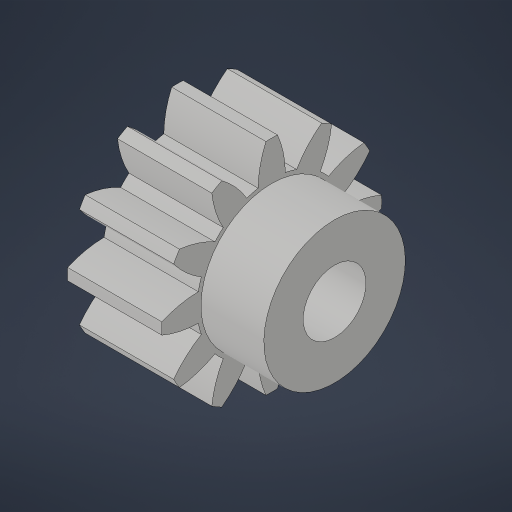
# Autodesk Inventor part: DS0.5-12_On
Saved by Autodesk Inventor 2024.2 (Build 282272000, 272)
## iProperties
Category: PARTsolutions
Company: KHK
Created: 2024-02-14
Part Number: DS0.5-12_On
Material: Generic
Catalog Web Link: www.cadenas.de
Description: Injection Molded Spur Gears (DS)-
Vendor: KHK
Document SubType Name: Modeling
Designer: psAdmin
Manufacturer: KHK
Mass: 0.117451 g
Surface Area: 2.6496 cm^2
Volume: 0.117451 cm^3
Density: 1 g/cm^3
Appearance: PSOLRGB-175-175-175
PSOL_IDENT_0: {$CADENAS_DATA/23d-libs/khk/spur_gears/injection_molded_spur_gears_ds.prj},190 {VTYP=3D},{NB=DS0.5-1
PSOL_IDENT_1: 2_On},{LINA=DS0.5-12},{NN=Injection Molded Spur Gears (DS)},{DATE=20.11.2023 06:40:42},{GEOMDATE=05.
PSOL_IDENT_2: 07.2019 08:33:51},{VERSION=},{LINEID=20},{WBVAR=TOOTH},{WBNUMERIC=}  {NB=DS0.5-12_On},{LINA=DS0.5-12
PSOL_IDENT_3: },{KT=DUMMY},{CN=DS0.5-12},{M=0.5},{MX=0.500},{Z=12},{A=2},{A1=4.0},{B=4.5},{B1=0.0},{C=6.0},{D=7.0}
PSOL_IDENT_4: ,{E=3},{F=4},{G=7},{H=0.0},{I=0.0},{J=0.6},{S=S8},{WMF=S8001.WMF},{VER=0},{TOOTH=On}
NB: DS0.5-12_On
NN: Injection Molded Spur Gears (DS)
NBSYN: $CN._$TOOTH.
LINA: DS0.5-12
CATALOG: KHK
CN: DS0.5-12
M: 0.5
Z: 12
A: 2
A1: 4
B: 4.5
B1: 0
C: 6
D: 7
E: 3
F: 4
G: 7
H: 0
I: 0
J: 0.6
S: S8
TOOTH: On
SUPPLIER: KHK
ARTICLENO: DS0.5-12_On
BOMINFO: DS0.5-12
CREATOR: CADENAS GmbH
Title: DS0.5-12
Author: Cadenas PARTsolutions
Autodesk Inventor part; units mm, degrees
ref_plane "YZ Plane" through (0, 0, 0) normal (1, 0, 0) x (0, 1, 0)
ref_plane "XZ Plane" through (0, 0, 0) normal (0, 1, 0) x (-1, 0, 0)
ref_plane "XY Plane" through (0, 0, 0) normal (0, 0, 1) x (1, 0, 0)
sketch "Sketch_8" plane through (0, 0, 0) normal (0, 0, 1) x (1, 0, 0)
  line L0 (7, 0) -> (0, 0)
  line L1 (0, 2) -> (0.6, 2)
  line L2 (0.6, 2) -> (0.6, 1)
  line L3 (0.6, 1) -> (5, 1)
  line L4 (5, 1) -> (5, 2.25)
  line L5 (5, 2.25) -> (3, 2.25)
  line L6 (3, 2.25) -> (3, 3.5)
  line L7 (3, 3.5) -> (0, 3.5)
  line L8 (0, 3.5) -> (0, 2)
  line L9 (0, -0.7) -> (0, 4.2) projected
  line L10 (-1.4, 0) -> (8.4, 0) projected
  dimension "d3" = 1.5
  dimension "d4" = 3
  dimension "d5" = 1
  dimension "d6" = 0.6
  dimension "d8" = 2
  dimension "d9" = 1.25
  dimension "d10" = 2
  constraints: 18 end point, 7 perpendicular, 3 point on line, 1 horizontal, 1 parallel
  measures "d3" distance of L7.end L1.start
  measures "d4" distance of L6.end L7.end
  measures "d5" distance of L1.end L2.end
  measures "d6" distance of L1.start L1.end
  measures "d8" distance of L0.end L1.start
  measures "d9" distance of L5.end L6.end
  measures "d10" distance of L4.end L5.end
revolve "Revolution1" add sketch "Sketch_8" angle 360 about axis through (7, 0, 0) along (1, 0, 0)
sketch "Sketch_5" plane through (0, 0, 0) normal (1, 0, 0) x (0, 1, 0)
  line L0 (7, 7) -> (-7, 7)
  line L1 (-7, 7) -> (-7, -7)
  line L2 (-7, -7) -> (7, -7)
  line L3 (7, -7) -> (7, 7)
  arc A0 (0.1832, 3.4952) -> (-0.1832, 3.4952) centre (0, 0) ccw
  arc A1 (-0.1832, 3.4952) -> (-0.4328, 2.3352) centre (2.5669, 2.2965) ccw
  arc A2 (-0.4328, 2.3352) -> (-0.7928, 2.2388) centre (0, 0) ccw
  arc A3 (-0.7928, 2.2388) -> (-1.589, 3.1185) centre (-3.3713, 0.7054) ccw
  arc A4 (-1.589, 3.1185) -> (-1.9062, 2.9353) centre (0, 0) ccw
  arc A5 (-1.9062, 2.9353) -> (-1.5424, 1.806) centre (1.0748, 3.2723) ccw
  arc A6 (-1.5424, 1.806) -> (-1.806, 1.5424) centre (0, 0) ccw
  arc A7 (-1.806, 1.5424) -> (-2.9353, 1.9062) centre (-3.2723, -1.0748) ccw
  arc A8 (-2.9353, 1.9062) -> (-3.1185, 1.589) centre (0, 0) ccw
  arc A9 (-3.1185, 1.589) -> (-2.2388, 0.7928) centre (-0.7054, 3.3713) ccw
  arc A10 (-2.2388, 0.7928) -> (-2.3352, 0.4328) centre (0, 0) ccw
  arc A11 (-2.3352, 0.4328) -> (-3.4952, 0.1832) centre (-2.2965, -2.5669) ccw
  arc A12 (-3.4952, 0.1832) -> (-3.4952, -0.1832) centre (0, 0) ccw
  arc A13 (-3.4952, -0.1832) -> (-2.3352, -0.4328) centre (-2.2965, 2.5669) ccw
  arc A14 (-2.3352, -0.4328) -> (-2.2388, -0.7928) centre (0, 0) ccw
  arc A15 (-2.2388, -0.7928) -> (-3.1185, -1.589) centre (-0.7054, -3.3713) ccw
  arc A16 (-3.1185, -1.589) -> (-2.9353, -1.9062) centre (0, 0) ccw
  arc A17 (-2.9353, -1.9062) -> (-1.806, -1.5424) centre (-3.2723, 1.0748) ccw
  arc A18 (-1.806, -1.5424) -> (-1.5424, -1.806) centre (0, 0) ccw
  arc A19 (-1.5424, -1.806) -> (-1.9062, -2.9353) centre (1.0748, -3.2723) ccw
  arc A20 (-1.9062, -2.9353) -> (-1.589, -3.1185) centre (0, 0) ccw
  arc A21 (-1.589, -3.1185) -> (-0.7928, -2.2388) centre (-3.3713, -0.7054) ccw
  arc A22 (-0.7928, -2.2388) -> (-0.4328, -2.3352) centre (0, 0) ccw
  arc A23 (-0.4328, -2.3352) -> (-0.1832, -3.4952) centre (2.5669, -2.2965) ccw
  arc A24 (-0.1832, -3.4952) -> (0.1832, -3.4952) centre (0, 0) ccw
  arc A25 (0.1832, -3.4952) -> (0.4328, -2.3352) centre (-2.5669, -2.2965) ccw
  arc A26 (0.4328, -2.3352) -> (0.7928, -2.2388) centre (0, 0) ccw
  arc A27 (0.7928, -2.2388) -> (1.589, -3.1185) centre (3.3713, -0.7054) ccw
  arc A28 (1.589, -3.1185) -> (1.9062, -2.9353) centre (0, 0) ccw
  arc A29 (1.9062, -2.9353) -> (1.5424, -1.806) centre (-1.0748, -3.2723) ccw
  arc A30 (1.5424, -1.806) -> (1.806, -1.5424) centre (0, 0) ccw
  arc A31 (1.806, -1.5424) -> (2.9353, -1.9062) centre (3.2723, 1.0748) ccw
  arc A32 (2.9353, -1.9062) -> (3.1185, -1.589) centre (0, 0) ccw
  arc A33 (3.1185, -1.589) -> (2.2388, -0.7928) centre (0.7054, -3.3713) ccw
  arc A34 (2.2388, -0.7928) -> (2.3352, -0.4328) centre (0, 0) ccw
  arc A35 (2.3352, -0.4328) -> (3.4952, -0.1832) centre (2.2965, 2.5669) ccw
  arc A36 (3.4952, -0.1832) -> (3.4952, 0.1832) centre (0, 0) ccw
  arc A37 (3.4952, 0.1832) -> (2.3352, 0.4328) centre (2.2965, -2.5669) ccw
  arc A38 (2.3352, 0.4328) -> (2.2388, 0.7928) centre (0, 0) ccw
  arc A39 (2.2388, 0.7928) -> (3.1185, 1.589) centre (0.7054, 3.3713) ccw
  arc A40 (3.1185, 1.589) -> (2.9353, 1.9062) centre (0, 0) ccw
  arc A41 (2.9353, 1.9062) -> (1.806, 1.5424) centre (3.2723, -1.0748) ccw
  arc A42 (1.806, 1.5424) -> (1.5424, 1.806) centre (0, 0) ccw
  arc A43 (1.5424, 1.806) -> (1.9062, 2.9353) centre (-1.0748, 3.2723) ccw
  arc A44 (1.9062, 2.9353) -> (1.589, 3.1185) centre (0, 0) ccw
  arc A45 (1.589, 3.1185) -> (0.7928, 2.2388) centre (3.3713, 0.7054) ccw
  arc A46 (0.7928, 2.2388) -> (0.4328, 2.3352) centre (0, 0) ccw
  arc A47 (0.4328, 2.3352) -> (0.1832, 3.4952) centre (-2.5669, 2.2965) ccw
  constraints: 96 point on circle, 48 centre point, 8 end point
extrude "Extrusion1" cut sketch "Sketch_5" along normal blind 3
body "Solid1"
